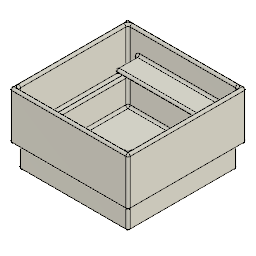
Filament Box Storage v2 (Autodesk Fusion 360 design; units mm, degrees)
Autodesk Fusion 360 part; units mm, degrees
sketch "Sketch1" plane through (0, 0, 0) normal (0, 0, 1) x (1, 0, 0)
  line L0 (13.0969, -13.0969) -> (-13.0969, -13.0969)
  line L1 (-13.0969, -13.0969) -> (-13.0969, 13.0969)
  line L2 (-13.0969, 13.0969) -> (13.0969, 13.0969)
  line L3 (13.0969, 13.0969) -> (13.0969, -13.0969)
  line L4 (13.0969, -13.0969) -> (-13.0969, 13.0969) construction
  line L5 (-13.0969, -13.0969) -> (13.0969, 13.0969) construction
  line L6 (12.0969, -12.0969) -> (-12.0969, -12.0969)
  line L7 (-12.0969, -12.0969) -> (-12.0969, 12.0969)
  line L8 (-12.0969, 12.0969) -> (12.0969, 12.0969)
  line L9 (12.0969, 12.0969) -> (12.0969, -12.0969)
  line L10 (-11.0969, -11.0969) -> (-11.0969, 11.0969)
  line L11 (-11.0969, 11.0969) -> (11.0969, 11.0969)
  line L12 (11.0969, 11.0969) -> (11.0969, -11.0969)
  line L13 (11.0969, -11.0969) -> (-11.0969, -11.0969)
  dimension "d7" = 26.1938
  dimension "d8" = 26.1938
  dimension "d10" = 1
  dimension "d18" = 2
  constraint horizontal L0
  constraint perpendicular L0 L1
  constraint parallel L0 L2
  constraint parallel L1 L3
  constraint coincident L4 origin
  constraint coincident L5 origin
  measures "d7" distance of L1.end L2.end
  measures "d8" distance of L0.end L1.end
extrude "Extrude1" add sketch "Sketch1" along normal blind 15.8083 contours L0 L1 L2 L3
extrude "Extrude2" add sketch "Sketch1" along normal blind 1 contours L6 L7 L8 L9 | L10 L11 L12 L13
extrude "Extrude3" [suppressed]
extrude "Extrude4" add sketch "Sketch1" along normal blind 7 contours L6 L7 L8 L9
extrude "Extrude5" cut sketch "Sketch1" along normal blind 5 contours L0 L1 L2 L3
sketch "Sketch2" plane through (0, 12.0969, 0) normal (0, -1, 0) x (1, 0, 0)
  line L0 (-12.0969, 7) -> (12.0969, 7)
  line L1 (12.0969, 7) -> (12.0969, 15.8083)
  line L2 (12.0969, 15.8083) -> (-12.0969, 15.8083)
  line L3 (-12.0969, 15.8083) -> (-12.0969, 7)
  line L4 (-10, 10.8083) -> (10, 10.8083)
  line L5 (10, 10.8083) -> (10, 9.8083)
  line L6 (10, 9.8083) -> (-10, 9.8083)
  line L7 (-10, 9.8083) -> (-10, 10.8083)
  line L8 (0, 15.8083) -> (0, 10.8083) construction
  point P0 (0, 10.8083)
  point P1 (0, 10.8083)
  dimension "d26" = 20
  dimension "d27" = 1
  dimension "d30" = 5
  constraint horizontal L4
  constraint vertical L5
  constraint horizontal L6
  constraint vertical L7
  constraint midpoint L4 P1
  constraint coincident P1 P0
  constraint midpoint L2 L8.start
  constraint perpendicular L2 L8
  measures "d26" distance of L4.start L4.end
  measures "d27" distance of L4.start L6.end
  measures "d30" distance of L8.start P1
extrude "Extrude6" add sketch "Sketch2" along normal blind 5 contours L4 L5 L6 L7
fillet "Fillet1" radius 0.4762 26 faces at (4.3656, -13.0969, 12.2056) (-12.0969, -4.0323, 9.9361) (-4.3656, 13.0969, 8.6028) (-4.0323, 4.0323, 0) (4.0323, -12.0969, 1.6667) (-13.0969, -4.3656, 8.6028) (3.699, -11.0969, 3) (-3.699, 3.699, 1) (-11.0969, -3.699, 3) (11.7635, 3.699, 7) (-12.7635, -4.0323, 15.8083) (-3.3333, 7.0969, 10.475) (-3.3333, 10.4302, 10.8083) (-12.7635, -4.0323, 5) (-3.699, 11.0969, 3) (3.3333, 12.0969, 14.1417) (11.0969, 3.699, 3) (3.3333, 10.4302, 9.8083) (13.0969, 4.3656, 8.6028) (12.0969, 4.0323, 1.6667) (4.0323, -12.0969, 9.9361) (-4.0323, 12.0969, 1.6667) (12.0969, 4.0323, 9.9361) (-10, 10.4302, 10.1417) (-12.0969, -4.0323, 1.6667) (10, 10.4302, 10.475)
equation "boxiw = 8.25 in"
equation "boxil = 8.25 in"
equation "cupnumw = 8"
equation "cupw = boxiw / cupnumw"
equation "cupl = boxil / cupnuml"
equation "cupnuml = 8"
equation "d7 = cupw"
equation "d8 = cupl"
equation "thick = 1 mm"
equation "d10 = thick"
equation "boxih = 2.75 in"
equation "cupnumh = 6"
equation "cuph = ( boxih + overlap * ( cupnumh - 1 ) ) / cupnumh"
equation "d14 = cuph"
equation "d16 = thick"
equation "d18 = thick * 2"
equation "d19 = mm"
equation "overlap = 5 mm"
equation "d22 = overlap + 2 * thick"
equation "d24 = overlap"
equation "d27 = thick"
equation "d30 = overlap"
equation "d32 = thick / 2.1"
